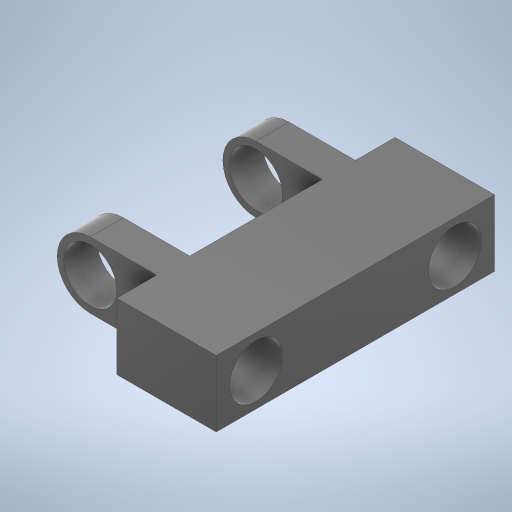
# Autodesk Inventor part: StabHalterSensor
Saved by Autodesk Inventor 2023 (Build 270158000, 158)
## iProperties
Created: 2024-01-25
Part Number: StabHalterSensor
Material: Generisch
Document SubType Name: Modeling
Designer: phili
Density: 1 g/cm^3
Appearance: Vorgabe
Author: phili
Autodesk Inventor part; units mm, degrees
ref_plane "YZ Plane" through (0, 0, 0) normal (1, 0, 0) x (0, 1, 0)
ref_plane "XZ Plane" through (0, 0, 0) normal (0, 1, 0) x (-1, 0, 0)
ref_plane "XY Plane" through (0, 0, 0) normal (0, 0, 1) x (1, 0, 0)
sketch "Skizze1" plane through (0, 0, 0) normal (1, 0, 0) x (0, 1, 0)
  line L0 (-5, -21) -> (5, -21)
  line L1 (5, -21) -> (5, 21)
  line L2 (5, 21) -> (-5, 21)
  line L3 (-5, 21) -> (-5, -21)
  line L4 (-5, -21) -> (5, 21) construction
  line L5 (5, -21) -> (-5, 21) construction
  point P0 (0, 0)
  dimension "d0" = 10
  dimension "d1" = 42
  constraints: 12 end point, 2 midpoint, 2 parallel, 1 horizontal, 1 perpendicular
  measures "d0" distance of L2.end L1.end
  measures "d1" distance of L1.end L0.end
extrude "Extrusion1" add sketch "Skizze1" along normal blind 15
sketch "Skizze2" plane through (15, 0, 0) normal (1, 0, 0) x (0, 0, -1)
  circle A0 centre (-15, 0) radius 4
  circle A1 centre (15, 0) radius 4
  point P0 (0, 0)
  dimension "d4" = 8
  dimension "d5" = 8
  dimension "d6" = 15
  dimension "d7" = 15
  constraints: 2 centre point
  measures "d4" diameter of A0
  measures "d5" diameter of A1
  measures "d6" distance of A0.centre point (0, 0)
  measures "d7" distance of A1.centre point (0, 0)
extrude "Extrusion2" cut sketch "Skizze2" against normal blind 10
sketch "Skizze3" plane through (0, 0, 0) normal (-1, 0, 0) x (0, 0, 1)
  line L0 (-21, 5) -> (21, 5) projected
  line L1 (21, -5) -> (-21, -5) projected
  line L2 (-15, 5) -> (-10, 5)
  line L3 (-10, 5) -> (-10, -5)
  line L4 (-10, -5) -> (-15, -5)
  line L5 (-15, -5) -> (-15, 5)
  line L6 (10, 5) -> (15, 5)
  line L7 (15, 5) -> (15, -5)
  line L8 (15, -5) -> (10, -5)
  line L9 (10, -5) -> (10, 5)
  point P0 (0, 0)
  dimension "d10" = 5
  dimension "d11" = 5
  dimension "d12" = 10
  dimension "d13" = 10
  constraints: 16 end point, 4 parallel, 4 point on line, 2 horizontal, 2 perpendicular
  measures "d10" distance of L3.end L4.end
  measures "d11" distance of L7.end L8.end
  measures "d12" distance from line of point (0, 0) L3
  measures "d13" distance from line of L9 point (0, 0)
extrude "Extrusion3" add sketch "Skizze3" along normal blind 15 contours L0 L3 L1 L5 | L0 L7 L1 L9
fillet "Rundung1" radius 5 4 edges at (-15, 5, -12.5) (-15, -5, -12.5) (-15, 5, 12.5) (-15, -5, 12.5)
sketch "Skizze4" plane through (0, -5, 15) normal (0, 0, 1) x (1, 0, 0)
  arc A0 (-10, 10) -> (-10, 0) centre (-10, 5) ccw projected
  circle A1 centre (-10, 5) radius 4
  point P0 (0, 5)
  dimension "d17" = 8
  constraints: 1 centre point, 1 coincident
  measures "d17" diameter of A1
extrude "Extrusion4" cut sketch "Skizze4" against normal through all
